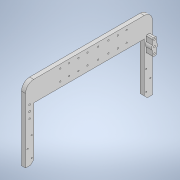
# Autodesk Inventor part: Frame
Saved by Autodesk Inventor 2020.1 (Build 241239000, 239)
## iProperties
Created: 2020-02-22
Part Number: Frame
Material: Generic
Document SubType Name: Modeling
Designer: Dominic
Density: 1 g/cm^3
Appearance: Default
Author: Dominic
Autodesk Inventor part; units mm, degrees
ref_plane "YZ Plane" through (0, 0, 0) normal (1, 0, 0) x (0, 1, 0)
ref_plane "XZ Plane" through (0, 0, 0) normal (0, 1, 0) x (-1, 0, 0)
ref_plane "XY Plane" through (0, 0, 0) normal (0, 0, 1) x (1, 0, 0)
sketch "Sketch1" plane through (0, 0, 0) normal (1, 0, 0) x (0, 1, 0)
  line L0 (0, 0) -> (45.3157, 0)
  line L1 (0, 172.72) -> (163.576, 172.72)
  line L2 (163.576, 172.72) -> (163.576, 198.12)
  line L3 (163.576, 198.12) -> (0, 198.12)
  line L4 (0, 198.12) -> (0, 172.72)
  dimension "d0" = 345.44
  dimension "d1" = 163.576
  dimension "d2" = 25.4
  constraints: 10 end point, 2 horizontal, 2 parallel, 1 perpendicular, 1 point on line
  measures "d0" diameter of L1 L0
  measures "d1" distance of L1.start L1.end
  measures "d2" distance of L1.end L2.end
extrude "Extrusion1" add sketch "Sketch1" along normal blind 12.7
sketch "Sketch3" plane through (12.7, 0, 0) normal (1, 0, 0) x (0, 0, -1)
  circle A0 centre (-185.42, 146.05) radius 3.175
  line L0 (-172.72, 0) -> (-172.72, 163.576) projected
  line L1 (-198.12, 0) -> (-172.72, 0) projected
  point P0 (0, 0)
  dimension "d10" = 6.35
  dimension "d11" = 12.7
  dimension "d62" = 146.05
  constraints: 1 centre point
  measures "d10" diameter of A0
  measures "d11" distance from line of L0 A0.centre
  measures "d62" distance from line of L1 A0.centre
extrude "Extrusion3" cut sketch "Sketch3" against normal blind 25.4
chamfer "Chamfer1" distance 9.525 angle 45 1 edges at (6.35, 0, 172.72)
sketch "Sketch4" plane through (12.7, 0, 0) normal (1, 0, 0) x (0, 0, -1)
  circle A0 centre (-185.42, 146.05) radius 3.175 projected
  circle A1 centre (-185.42, 146.05) radius 9.525
  point P0 (0, 0)
  dimension "d18" = 19.05
  constraints: 1 centre point, 1 coincident
  measures "d18" diameter of A1
extrude "Extrusion4" add sketch "Sketch4" along normal blind 19.05
mirror "Mirror2" about plane through (0, 0, 0) normal (0, 0, 1) of "Extrusion1", "Extrusion3", "Chamfer1", "Extrusion4"
sketch "Sketch5" plane through (0, 0, 0) normal (-1, 0, 0) x (0, 0, 1)
  line L0 (172.72, 163.576) -> (198.12, 163.576) projected
  line L1 (198.12, 163.576) -> (-198.12, 163.576)
  line L2 (-198.12, 163.576) -> (-198.12, 227.076)
  line L3 (-198.12, 227.076) -> (198.12, 227.076)
  line L4 (198.12, 227.076) -> (198.12, 163.576)
  point P0 (0, 0)
  dimension "d21" = 63.5
  constraints: 8 end point, 2 parallel, 1 coincident, 1 horizontal, 1 perpendicular
  measures "d21" distance of L1.end L2.end
extrude "Extrusion5" add sketch "Sketch5" against normal up to surface (12.7 mm away)
fillet "Fillet2" radius 25.4 2 edges at (6.35, 227.076, 198.12) (6.35, 227.076, -198.12)
sketch "Sketch6" plane through (12.7, 0, 0) normal (1, 0, 0) x (0, 0, -1)
  line L0 (188.595, 120.65) -> (182.245, 120.65)
  line L1 (179.07, 123.825) -> (179.07, 168.275)
  line L2 (182.245, 171.45) -> (188.595, 171.45)
  line L3 (191.77, 168.275) -> (191.77, 123.825)
  circle A0 centre (185.42, 146.05) radius 3.175 projected
  line L4 (191.77, 120.65) -> (179.07, 171.45) construction
  line L5 (179.07, 120.65) -> (191.77, 171.45) construction
  arc A1 (182.245, 171.45) -> (179.07, 168.275) centre (182.245, 168.275) ccw
  arc A2 (191.77, 168.275) -> (188.595, 171.45) centre (188.595, 168.275) ccw
  arc A3 (188.595, 120.65) -> (191.77, 123.825) centre (188.595, 123.825) ccw
  arc A4 (179.07, 123.825) -> (182.245, 120.65) centre (182.245, 123.825) ccw
  circle A5 centre (185.42, 146.05) radius 9.525 projected
  circle A6 centre (185.42, 165.1) radius 2.6289
  line L6 (185.42, 165.1) -> (185.42, 171.45)
  circle A7 centre (185.42, 127) radius 2.6289
  line L7 (185.42, 127) -> (185.42, 120.65)
  point P0 (0, 0)
  point P1 (191.77, 138.9505)
  point P2 (179.07, 138.9505)
  point P3 (179.07, 153.1495)
  point P4 (191.77, 153.1495)
  dimension "d25" = 12.7
  dimension "d26" = 50.8
  dimension "d27" = 3.175
  dimension "d28" = 5.2578
  dimension "d29" = 6.35
  dimension "d30" = 5.2578
  dimension "d31" = 6.35
  constraints: 16 end point, 8 point on circle, 8 point on line, 8 tangent, 6 centre point, 4 midpoint, 3 equal radius, 2 parallel, 2 vertical, 1 horizontal, 1 perpendicular
  measures "d25" distance of L4.end L5.end
  measures "d26" distance of L5.start L4.end
  measures "d27" radius of A1
  measures "d28" diameter of A6
  measures "d29" distance of L6.start L6.end
  measures "d30" diameter of A7
  measures "d31" distance of L7.start L7.end
extrude "Extrusion6" add sketch "Sketch6" along normal blind 19.05 contours L0 A4 L1 A5 L3 A3 | A5 L1 A1 L2 A2 L3
sketch "Sketch9" plane through (0, 227.076, 172.72) normal (0, 1, 0) x (1, 0, 0)
  line L0 (0, 345.44) -> (0, 0) projected
  line L1 (0, 228.6) -> (6.35, 228.6)
  line L2 (6.35, 228.6) -> (6.35, 116.84)
  line L3 (6.35, 116.84) -> (12.7, 116.84)
  line L4 (12.7, 345.44) -> (12.7, 0) projected
  line L5 (0, -25.4) -> (12.7, -25.4) projected
  point P0 (0, 172.72)
  point P1 (6.35, 172.72)
  point P2 (0, 172.72)
  dimension "d47" = 6.35
  dimension "d48" = 254
  constraints: 6 end point, 2 midpoint, 2 perpendicular, 2 point on line, 1 horizontal alignment, 1 parallel
  measures "d47" distance of L1.start L1.end
  measures "d48" distance between parallel lines of L5 L1
sketch "Sketch10" plane through (12.7, 0, 0) normal (1, 0, 0) x (0, 0, -1)
  circle A0 centre (179.07, 17.4625) radius 2.0828
  circle A1 centre (191.77, 48.4187) radius 2.0828
  circle A2 centre (179.07, 79.375) radius 2.0828
  line L0 (185.42, 0) -> (198.12, 0)
  line L1 (198.12, 88.9) -> (198.12, 0)
  line L2 (172.72, 88.9) -> (198.12, 88.9)
  line L3 (172.72, 88.9) -> (172.72, 12.7)
  line L4 (172.72, 12.7) -> (185.42, 0)
  point P0 (0, 0)
  point P1 (-12.7, 88.9)
  dimension "d49" = 6.35
  dimension "d50" = 9.525
  dimension "d51" = 25.4
  dimension "d52" = 76.2
  dimension "d53" = 88.9
  dimension "d54" = 12.7
  dimension "d55" = 4.7625
  dimension "d56" = 6.35
  dimension "d57" = 19.05
  dimension "d58" = 40.4813
  dimension "d59" = 4.1656
  constraints: 10 end point, 3 centre point, 3 perpendicular, 2 equal radius, 1 coincident, 1 horizontal
  measures "d49" distance from line of L3 A2.centre
  measures "d50" distance from line of L2 A2.centre
  measures "d51" distance of L2.start L1.start
  measures "d52" distance of L2.start L3.end
  measures "d53" distance of L1.start L0.end
  measures "d54" distance of L0.start L0.end
  measures "d55" vertical distance of L3.end A0.centre
  measures "d56" distance from line of L3 A0.centre
  measures "d57" distance from line of L3 A1.centre
  measures "d58" distance from line of L2 A1.centre
  measures "d59" diameter of A2
extrude "Extrusion8" cut sketch "Sketch10" against normal through all contours A0 | A1 | A2
mirror "Mirror3" about plane through (0, 0, 0) normal (0, 0, 1) of "Extrusion8"
sketch "Sketch11" plane through (31.75, 146.05, 185.42) normal (1, 0, 0) x (0, 0, -1)
  circle A0 centre (0, 0) radius 9.525 projected
  circle A1 centre (0, 0) radius 3.175 projected
  point P0 (185.42, -146.05)
extrude "Extrusion9" cut sketch "Sketch11" against normal up to surface (19.05 mm away)
sketch "Sketch12" plane through (12.7, 0, 0) normal (1, 0, 0) x (0, 0, -1)
  circle A0 centre (-185.42, 146.05) radius 3.175 projected
  line L0 (-185.42, 165.1) -> (-185.42, 127)
  circle A1 centre (-185.42, 165.1) radius 2.6035
  circle A2 centre (-185.42, 127) radius 2.6035
  point P0 (0, 0)
  dimension "d65" = 38.1
  dimension "d66" = 5.207
  dimension "d67" = 5.207
  constraints: 3 coincident, 2 centre point, 2 end point, 1 midpoint, 1 vertical
  measures "d65" distance of L0.start L0.end
  measures "d66" diameter of A1
  measures "d67" diameter of A2
extrude "Extrusion10" cut sketch "Sketch12" against normal blind 25.4 contours A2 | A1
sketch "Sketch13" plane through (0, 0, 0) normal (-1, 0, 0) x (0, 0, 1)
  line L0 (-60.6806, 180.6448) -> (-117.602, 180.6448)
  line L1 (-117.602, 180.6448) -> (-117.602, 215.5698)
  line L2 (-117.602, 215.5698) -> (-60.6806, 215.5698)
  line L3 (-60.6806, 215.5698) -> (-60.6806, 180.6448)
  line L4 (-60.6806, 180.6448) -> (-117.602, 215.5698) construction
  line L5 (-117.602, 180.6448) -> (-60.6806, 215.5698) construction
  line L6 (-198.12, 201.676) -> (-198.12, 0) projected
  line L7 (-90.0938, 214.5284) -> (-90.0938, 179.6034)
  line L8 (172.72, 227.076) -> (-172.72, 227.076) projected
  line L9 (-90.0938, 214.5284) -> (-28.448, 214.5284)
  line L10 (-28.448, 214.5284) -> (-28.448, 179.6034)
  line L11 (-28.448, 179.6034) -> (-90.0938, 179.6034)
  line L12 (-90.0938, 179.6034) -> (-90.0938, 214.5284)
  line L13 (-60.6806, 215.5698) -> (4.6736, 215.5698)
  line L14 (4.6736, 215.5698) -> (4.6736, 180.6448)
  line L15 (4.6736, 180.6448) -> (-60.6806, 180.6448)
  line L16 (-60.6806, 180.6448) -> (-60.6806, 215.5698)
  line L17 (-28.448, 214.5284) -> (33.02, 214.5284)
  line L18 (33.02, 214.5284) -> (33.02, 179.6034)
  line L19 (33.02, 179.6034) -> (-28.448, 179.6034)
  line L20 (-28.448, 179.6034) -> (-28.448, 214.5284)
  line L21 (4.6736, 180.6448) -> (62.2808, 180.6448)
  line L22 (62.2808, 180.6448) -> (62.2808, 215.5698)
  line L23 (62.2808, 215.5698) -> (4.6736, 215.5698)
  line L24 (4.6736, 215.5698) -> (4.6736, 180.6448)
  line L25 (33.02, 214.5284) -> (89.535, 214.5284)
  line L26 (89.535, 214.5284) -> (89.535, 179.6034)
  line L27 (89.535, 179.6034) -> (33.02, 179.6034)
  line L28 (33.02, 179.6034) -> (33.02, 214.5284)
  point P0 (0, 0)
  point P1 (-89.1413, 198.1073)
  point P2 (-89.1413, 198.1073)
  dimension "d71" = 80.518
  dimension "d72" = 34.925
  dimension "d74" = 1.0414
  dimension "d75" = 27.5082
  dimension "d76" = 56.9214
  dimension "d77" = 11.5062
  dimension "d78" = 89.154
  dimension "d79" = 65.3542
  dimension "d80" = 61.468
  dimension "d81" = 57.6072
  dimension "d82" = 56.515
  constraints: 54 end point, 13 parallel, 6 horizontal, 6 perpendicular, 3 midpoint, 1 vertical
  measures "d71" distance between parallel lines of L6 L1
  measures "d72" distance of L0.end L1.end
  measures "d74" distance from line of L2 L7.start
  measures "d75" distance between parallel lines of L1 L7
  measures "d76" distance of L1.end L2.end
  measures "d77" distance between parallel lines of L8 L2
  measures "d78" distance between parallel lines of L10 L1
  measures "d79" distance of L2.end L13.end
  measures "d80" distance of L18.end L10.end
  measures "d81" distance of L22.end L13.end
  measures "d82" distance of L17.end L25.end
hole "Hole1" at (0, 215.5698, -117.602) at (0, 180.6448, -117.602) at (0, 214.5284, -90.0938) at (0, 179.6034, -90.0938) at (0, 180.6448, -60.6806) at (0, 215.5698, -60.6806) at (0, 214.5284, -28.448) at (0, 179.6034, -28.448) at (0, 215.5698, 4.6736) at (0, 180.6448, 4.6736) at (0, 214.5284, 33.02) at (0, 179.6034, 33.02) at (0, 215.5698, 62.2808) at (0, 180.6448, 62.2808) at (0, 179.6034, 89.535) at (0, 214.5284, 89.535) direction (1, 0, 0) diameter 4.445 end through all
sketch "Sketch14" plane through (0, 227.076, 172.72) normal (0, 1, 0) x (1, 0, 0)
  line L0 (0, 345.44) -> (0, 0) projected
  line L1 (6.35, 245.745) -> (6.35, 99.695)
  line L2 (12.7, 345.44) -> (12.7, 0) projected
  line L3 (6.35, 99.695) -> (0, 99.695)
  line L4 (0, 0) -> (0, 345.44) projected
  line L5 (6.35, 245.745) -> (12.7, 245.745)
  point P0 (0, 172.72)
  point P1 (6.35, 172.72)
  point P2 (0, 172.72)
  dimension "d90" = 146.05
  constraints: 6 end point, 2 midpoint, 2 perpendicular, 2 point on line, 1 horizontal alignment, 1 parallel, 1 vertical
  measures "d90" distance of L1.start L1.end
equation "\"d30\" = d28"
equation "\"d31\" = d29"
body "Solid1"
